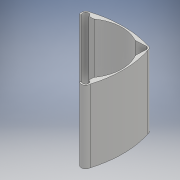
# Autodesk Inventor part: Cage60mm-2sides-InnerD74mm-L75mm
Saved by Autodesk Inventor 2017 (Build 210142000, 142)
## iProperties
Created: 2022-04-01
Part Number: Cage60mm-2sides-InnerD74mm-L75mm
Material: Generic
Document SubType Name: Modeling
Designer: Nikita
Density: 1 g/cm^3
Appearance: Default
Author: Nikita
Autodesk Inventor part; units mm, degrees
ref_plane "YZ Plane" through (0, 0, 0) normal (1, 0, 0) x (0, 1, 0)
ref_plane "XZ Plane" through (0, 0, 0) normal (0, 1, 0) x (-1, 0, 0)
ref_plane "XY Plane" through (0, 0, 0) normal (0, 0, 1) x (1, 0, 0)
sketch "Sketch1" plane through (0, 0, 0) normal (0, 0, 1) x (1, 0, 0)
  arc A0 (32.6355, 29.9298) -> (29.3759, 33.1607) centre (29.5384, 30.0649) ccw
  arc A1 (27.8274, -32.2191) -> (30.1546, -26.93) centre (30.0194, -30.0271) ccw
  arc A2 (32.4933, 26.671) -> (34.0351, 30.2371) centre (29.5384, 30.0649) ccw
  arc A3 (26.8375, -33.2091) -> (34.5127, -29.7804) centre (30.0194, -30.0271) ccw
  line L0 (-29.9673, 30.0452) -> (-33.1472, 26.8653)
  line L1 (-29.9673, 30.0452) -> (-25.4702, 30.0452) construction
  line L2 (-29.9673, 30.0452) -> (-21.8579, 30.471)
  line L3 (30.0194, -30.0271) -> (30.3698, -21.9984)
  line L4 (30.0194, -30.0271) -> (26.8375, -33.2091)
  circle A4 centre (0, 0) radius 37.5
  arc A5 (34.5127, -29.7804) -> (34.0351, 30.2371) centre (-61.1139, -0.5306) ccw
  arc A6 (29.3158, 34.5594) -> (-29.9754, 34.5423) centre (-0.3022, -60.9538) ccw
  line L5 (18.5473, 32.5922) -> (29.3759, 33.1607)
  line L6 (32.1704, 19.2696) -> (32.6355, 29.9298)
  arc A7 (29.3158, 34.5594) -> (26.1185, 32.9896) centre (29.5384, 30.0649) ccw
  arc A8 (34.0351, 30.2371) -> (29.3158, 34.5594) centre (29.5384, 30.0649) ccw
  arc A9 (-29.9754, 34.5423) -> (-33.1472, 26.8653) centre (-29.9673, 30.0452) ccw
  arc A10 (-26.8454, 30.2091) -> (-32.1778, 27.8347) centre (-29.9673, 30.0452) ccw
  dimension "d0" = 6.2
  dimension "d1" = 6.2
  dimension "d6" = 9
  dimension "d7" = 9
  dimension "d8" = 135
  dimension "d9" = 75
  dimension "d11" = 100
  dimension "d12" = 100
  constraints: 25 point on circle, 14 end point, 11 centre point, 8 point on line, 4 coincident, 4 tangent, 1 equal length, 1 horizontal
  measures "d0" diameter of A0
  measures "d1" diameter of A1
  measures "d6" diameter of A2
  measures "d7" diameter of A3
  measures "d8" angle of L0 L1
  measures "d9" diameter of A4
  measures "d11" radius of A5
  measures "d12" radius of A6
extrude "Extrusion1" add sketch "Sketch1" along normal blind 75 contours A0 L5 A7 A8 A2 L6 | A2 A5 A3 L4 A1 L3 A4 L6 | L5 A4 L2 A10 L0 A9 A6 A7
body "Solid1"
